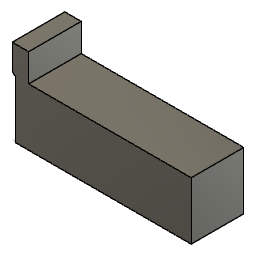
SumoPruebaV7 v1 (Autodesk Fusion 360 archive; units mm, degrees)
design "bateria"
Autodesk Fusion 360 part; units mm, degrees
sketch "Boceto1" plane through (0, 0, 0) normal (0, 1, 0) x (1, 0, 0)
  line L0 (53.5, 16) -> (-53.5, 16)
  line L1 (-53.5, 16) -> (-53.5, -16)
  line L2 (-53.5, -16) -> (53.5, -16)
  line L3 (53.5, -16) -> (53.5, 16)
  line L4 (53.5, 16) -> (-53.5, -16) construction
  line L5 (-53.5, 16) -> (53.5, -16) construction
  dimension "d1" = 107
  dimension "d2" = 32
  constraint horizontal L0
  constraint perpendicular L0 L1
  constraint parallel L0 L2
  constraint parallel L1 L3
  constraint coincident L4 origin
  constraint coincident L5 origin
  measures "d1" distance of L1.end L2.end
  measures "d2" distance of L0.end L1.end
extrude "Extruir1" add sketch "Boceto1" along normal blind 35
sketch "Boceto2" plane through (0, 35, 0) normal (0, 1, 0) x (-1, 0, 0)
  line L0 (-53.5, 16) -> (-53.5, -16)
  line L1 (-53.5, -16) -> (53.5, -16)
  line L2 (53.5, -16) -> (53.5, 16)
  line L3 (53.5, 16) -> (-53.5, 16)
  line L4 (53.5, 16) -> (55.5, 16)
  line L5 (55.5, 16) -> (55.5, -16)
  line L6 (55.5, -16) -> (53.5, -16)
  line L7 (45.5, 16) -> (45.5, -16)
  dimension "d5" = 8
  dimension "d6" = 2
  constraint coincident L2.end L3.start
  constraint perpendicular L2 L4
  constraint perpendicular L4 L5
  constraint coincident L1.end L2.start
  constraint collinear L1 L6
  constraint coincident L3 L7.start
  constraint coincident L1 L7.end
  constraint perpendicular L1 L7
  measures "d5" distance of L2 L7
  measures "d6" distance of L2 L5
extrude "Extruir2" add sketch "Boceto2" along normal blind 17 contours L1 L2 L3 L7 | L2 L4 L5 L6
fillet "Empalme1" radius 3 1 edges at (-55.5, 35, 0)

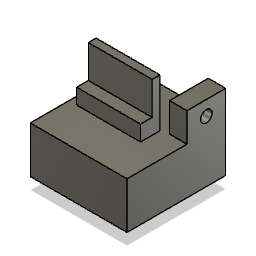
design "SensorIRteo"
Autodesk Fusion 360 part; units mm, degrees
sketch "Boceto1" plane through (0, 0, 0) normal (0, 0, 1) x (1, 0, 0)
  line L0 (8.25, 13.75) -> (-8.25, 13.75)
  line L1 (-8.25, 13.75) -> (-8.25, -13.75)
  line L2 (-8.25, -13.75) -> (8.25, -13.75)
  line L3 (8.25, -13.75) -> (8.25, 13.75)
  line L4 (8.25, 13.75) -> (-8.25, -13.75) construction
  line L5 (-8.25, 13.75) -> (8.25, -13.75) construction
  line L6 (-10.25, -10.75) -> (14.75, -10.75)
  line L7 (14.75, -10.75) -> (14.75, 1.25)
  line L8 (14.75, 1.25) -> (-10.25, 1.25)
  line L9 (-10.25, 1.25) -> (-10.25, -10.75)
  line L10 (14.75, 1.25) -> (14.75, 8.75)
  line L11 (14.75, 8.75) -> (10.25, 8.75)
  line L12 (10.25, 8.75) -> (10.25, 1.25)
  line L13 (-8.25, 5.25) -> (8.25, 5.25)
  dimension "d1" = 16.5
  dimension "d2" = 27.5
  dimension "d3" = 3
  dimension "d4" = 12
  dimension "d5" = 6.5
  dimension "d6" = 2
  dimension "d7" = 4.5
  dimension "d8" = 7.5
  dimension "d28" = 8.5
  constraint horizontal L0
  constraint perpendicular L0 L1
  constraint parallel L0 L2
  constraint parallel L1 L3
  constraint coincident L4 origin
  constraint coincident L5 origin
  constraint perpendicular L3 L6
  constraint perpendicular L6 L7
  constraint perpendicular L1 L8
  constraint perpendicular L8 L9
  constraint perpendicular L8 L10
  constraint perpendicular L7 L11
  constraint coincident L8 L12.end
  constraint perpendicular L8 L12
  constraint coincident L1 L13.start
  constraint coincident L3 L13.end
  constraint perpendicular L3 L13
  measures "d1" distance of L1.end L2.end
  measures "d2" distance of L0.end L1.end
  measures "d3" distance of L2 L6
  measures "d4" distance of L6 L8
  measures "d5" distance of L3 L7
  measures "d6" distance of L1 L9
  measures "d7" distance of L10 L12
  measures "d8" distance of L8 L11
  measures "d28" distance of L0 L13
extrude "Extruir1" add sketch "Boceto1" along normal blind 2 contours L0 L1 L3 L13 | L1 L3 L8 L13 | L1 L3 L6 L8 | L1 L2 L3 L6
extrude "Extruir2" add sketch "Boceto1" against normal blind 10.5 contours L1 L3 L6 L8
extrude "Extruir3" add sketch "Boceto1" along normal blind 13 from surface at 2 contours L1 L3 L6 L8
extrude "Extruir4" add sketch "Boceto1" along normal up to surface (25.5 mm away) from surface at -10.5 contours L3 L6 L7 L8 | L1 L6 L8 L9
extrude "Extruir5" add sketch "Boceto1" along normal blind 10 from surface at -10.5 contours L8 L10 L11 L12
sketch "Boceto2" plane through (14.75, 0, 0) normal (1, 0, 0) x (0, 0, -1)
  line L0 (-15, 1.25) -> (-15, -10.75)
  line L1 (-15, -10.75) -> (10.5, -10.75)
  line L2 (10.5, -10.75) -> (10.5, 8.75)
  line L3 (10.5, 8.75) -> (0.5, 8.75)
  line L4 (0.5, 8.75) -> (0.5, 1.25)
  line L5 (0.5, 1.25) -> (-15, 1.25)
  line L6 (-2, 1.25) -> (0, 1.25)
  line L7 (0, 1.25) -> (0, 13.75)
  line L8 (0, 13.75) -> (-2, 13.75)
  line L9 (-2, 13.75) -> (-2, 1.25)
  circle A0 centre (5.5, 5) radius 1.5
  dimension "d23" = 3
  dimension "d24" = 3.75
  dimension "d25" = 5
  measures "d23" diameter of A0
  measures "d24" distance of L3 A0.centre
  measures "d25" distance of L4 A0.centre
extrude "Extruir6" cut sketch "Boceto2" against normal up to surface (4.5 mm away) contours A0
extrude "Extruir7" add sketch "Boceto1" along normal blind 3 from surface at 2 contours L1 L3 L8 L13
named bodies: "cuerpo1"

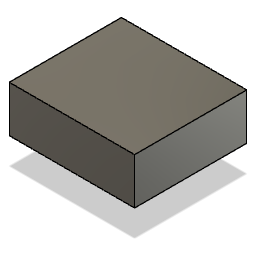
design "placaLeds"
Autodesk Fusion 360 part; units mm, degrees
sketch "Boceto1" plane through (0, 0, 0) normal (0, 1, 0) x (1, 0, 0)
  line L0 (19, 17) -> (-19, 17)
  line L1 (-19, 17) -> (-19, -17)
  line L2 (-19, -17) -> (19, -17)
  line L3 (19, -17) -> (19, 17)
  line L4 (19, 17) -> (-19, -17) construction
  line L5 (-19, 17) -> (19, -17) construction
  line L6 (-5.5, 13) -> (10, 13)
  line L7 (10, 13) -> (10, 10.5)
  line L8 (10, 10.5) -> (-5.5, 10.5)
  line L9 (-5.5, 10.5) -> (-5.5, 13)
  dimension "d1" = 38
  dimension "d2" = 34
  dimension "d3" = 4
  dimension "d4" = 2.5
  dimension "d5" = 9
  dimension "d6" = 13.5
  constraint horizontal L0
  constraint perpendicular L0 L1
  constraint parallel L0 L2
  constraint parallel L1 L3
  constraint coincident L4 origin
  constraint coincident L5 origin
  constraint perpendicular L1 L6
  constraint perpendicular L6 L7
  constraint perpendicular L1 L8
  constraint perpendicular L6 L9
  measures "d1" distance of L1.end L2.end
  measures "d2" distance of L0.end L1.end
  measures "d3" distance of L0 L6
  measures "d4" distance of L6 L8
  measures "d5" distance of L3 L7
  measures "d6" distance of L1 L9
extrude "Extruir1" add sketch "Boceto1" along normal blind 14 contours L0 L1 L2 L3 | L6 L7 L8 L9
extrude "Extruir2" add sketch "Boceto1" against normal blind 8 contours L6 L7 L8 L9
